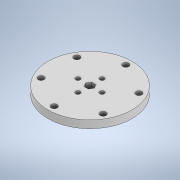
# Autodesk Inventor part: WheelMount_v2_vCAD
Saved by Autodesk Inventor 2020.2 (Build 242310000, 310)
## iProperties
Created: 2020-01-14
Part Number: WheelMount_v2_vCAD
Material: Generic
Document SubType Name: Modeling
Designer: maple
Density: 1 g/cm^3
Appearance: Default
Author: maple
Autodesk Inventor part; units mm, degrees
ref_plane "YZ Plane" through (0, 0, 0) normal (1, 0, 0) x (0, 1, 0)
ref_plane "XZ Plane" through (0, 0, 0) normal (0, 1, 0) x (-1, 0, 0)
ref_plane "XY Plane" through (0, 0, 0) normal (0, 0, 1) x (1, 0, 0)
sketch "Sketch1" plane through (0, 0, 0) normal (0, 1, 0) x (-1, 0, 0)
  circle A0 centre (0, 0) radius 27.94
  dimension "d0" = 55.88
  constraints: 1 centre point, 1 coincident
  measures "d0" diameter of A0
extrude "Extrusion1" add sketch "Sketch1" along normal blind 5.08
sketch "Sketch12" plane through (0, 5.08, 0) normal (0, 1, 0) x (1, 0, 0)
  circle A0 centre (0, 0) radius 27.94 projected
  line L0 (2.9329, 0) -> (1.4665, -2.54)
  line L1 (1.4665, -2.54) -> (-1.4665, -2.54)
  line L2 (-1.4665, -2.54) -> (-2.9329, 0)
  line L3 (-2.9329, 0) -> (-1.4665, 2.54)
  line L4 (-1.4665, 2.54) -> (1.4665, 2.54)
  line L5 (1.4665, 2.54) -> (2.9329, 0)
  dimension "d33" = 5.08
  constraints: 12 end point, 1 coincident, 1 horizontal, 13 other
  measures "d33" distance between parallel lines of L1 L4
extrude "Extrusion9" cut sketch "Sketch12" against normal blind 25.4 contours L0 L1 L2 L3 L4 L5
sketch "Sketch6" plane through (0, 5.08, 0) normal (0, 1, 0) x (1, 0, 0)
  circle A0 centre (0, 23.8125) radius 1.9939
  circle A1 centre (20.6222, 11.9063) radius 1.9939
  circle A2 centre (20.6222, -11.9063) radius 1.9939
  circle A3 centre (0, -23.8125) radius 1.9939
  circle A4 centre (-20.6222, -11.9063) radius 1.9939
  circle A5 centre (-20.6222, 11.9063) radius 1.9939
  point P0 (0, 0)
  point P1 (0, 0)
  constraints: 6 centre point
extrude "Extrusion5" cut sketch "Sketch6" against normal blind 25.4
sketch "Sketch13" plane through (0, 5.08, 0) normal (0, 1, 0) x (1, 0, 0)
  circle A0 centre (0, 8.001) radius 1.524
  point P0 (0, 0)
  dimension "d42" = 0
  dimension "d43" = 8.001
  dimension "d44" = 3.048
  constraints: 1 centre point
  measures "d42" horizontal distance of point (0, 0) A0.centre
  measures "d43" distance of point (0, 0) A0.centre
  measures "d44" diameter of A0
extrude "Extrusion10" cut sketch "Sketch13" against normal blind 25.4
pattern_circular "Circular Pattern4" count 4 over 360 about axis through (0, 0, 0) along (0, 1, 0) of "Extrusion10"
body "Solid1"
